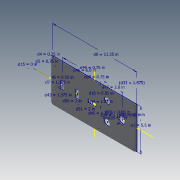
# Autodesk Inventor part: FLUGGER SWITCH PANEL
Saved by Autodesk Inventor 2020.3 (Build 243373000, 373)
## iProperties
RuleStatus: InUse
AfterDocSave0: file://Part Number Cleaner
Created: 2020-01-25
Material: Generic
Vendor: HHMI: JRC - ID&F
Document SubType Name: Modeling
Designer: arnoldj
Density: 1 g/cm^3
Appearance: Default
DESIGN DEPARTMENT: HHMI: JRC - ID&F
ALTERED ITEM PART NUMBER: N/A
ALTERED ITEM VENDOR: N/A
ALTERED ITEM DESCRIPTION: N/A
Author: arnoldj
Revision Number: 0
Autodesk Inventor part; units mm, degrees
ref_plane "YZ Plane" through (0, 0, 0) normal (1, 0, 0) x (0, 1, 0)
ref_plane "XZ Plane" through (0, 0, 0) normal (0, 1, 0) x (-1, 0, 0)
ref_plane "XY Plane" through (0, 0, 0) normal (0, 0, 1) x (1, 0, 0)
sketch "Sketch1" plane through (0, 0, 0) normal (0, 0, 1) x (1, 0, 0)
  line L0 (0, 97.79) -> (0, -97.79) projected
  line L1 (-200.025, 0) -> (200.025, 0) projected
  line L2 (142.875, -69.85) -> (-142.875, -69.85)
  line L3 (-142.875, -69.85) -> (-142.875, 69.85)
  line L4 (-142.875, 69.85) -> (142.875, 69.85)
  line L5 (142.875, 69.85) -> (142.875, -69.85)
  line L6 (142.875, -69.85) -> (-142.875, 69.85) construction
  line L7 (-142.875, -69.85) -> (142.875, 69.85) construction
  line L8 (-136.525, -63.5) -> (136.525, -63.5) construction
  line L9 (136.525, -63.5) -> (136.525, 63.5) construction
  line L10 (136.525, 63.5) -> (-136.525, 63.5) construction
  line L11 (-136.525, 63.5) -> (-136.525, -63.5) construction
  line L12 (-136.525, -63.5) -> (136.525, 63.5) construction
  line L13 (136.525, -63.5) -> (-136.525, 63.5) construction
  line L14 (-100.965, -14.2875) -> (-114.935, -14.2875)
  line L15 (-114.935, -14.2875) -> (-114.935, 14.2875)
  line L16 (-114.935, 14.2875) -> (-100.965, 14.2875)
  line L17 (-100.965, 14.2875) -> (-100.965, -14.2875)
  line L18 (-100.965, -14.2875) -> (-114.935, 14.2875) construction
  line L19 (-114.935, -14.2875) -> (-100.965, 14.2875) construction
  circle A0 centre (44.45, 31.75) radius 10.795
  circle A1 centre (44.45, -31.75) radius 10.795
  circle A2 centre (95.25, 0) radius 11.303
  circle A3 centre (95.25, 0) radius 30 construction
  line L20 (-64.135, -14.2875) -> (-50.165, -14.2875)
  line L21 (-50.165, -14.2875) -> (-50.165, 14.2875)
  line L22 (-50.165, 14.2875) -> (-64.135, 14.2875)
  line L23 (-64.135, 14.2875) -> (-64.135, -14.2875)
  line L24 (-64.135, -14.2875) -> (-50.165, 14.2875) construction
  line L25 (-50.165, -14.2875) -> (-64.135, 14.2875) construction
  line L26 (7.9375, -6.985) -> (-20.6375, -6.985)
  line L27 (-20.6375, -6.985) -> (-20.6375, 6.985)
  line L28 (-20.6375, 6.985) -> (7.9375, 6.985)
  line L29 (7.9375, 6.985) -> (7.9375, -6.985)
  line L30 (7.9375, -6.985) -> (-20.6375, 6.985) construction
  line L31 (-20.6375, -6.985) -> (7.9375, 6.985) construction
  point P0 (0, 0)
  point P1 (-107.95, 0)
  point P2 (95.25, 14.732)
  point P3 (95.25, -14.732)
  point P4 (-19.05, 63.5)
  point P5 (-19.05, -63.5)
  point P6 (19.05, -63.5)
  point P7 (19.05, 63.5)
  point P8 (-57.15, 0)
  point P9 (-6.35, 0)
  dimension "d0" = 285.75
  dimension "d1" = 139.7
  dimension "d4" = 6.35
  dimension "d5" = 6.35
  dimension "d6" = 13.97
  dimension "d7" = 28.575
  dimension "d15" = 0
  dimension "d16" = 21.59
  dimension "d20" = 22.606
  dimension "d22" = 60
  dimension "d33" = 47.625
  dimension "d34" = 14.732
  dimension "d35" = 14.732
  dimension "d43" = 34.925
  dimension "d44" = 31.75
  dimension "d45" = 31.75
  dimension "d46" = 152.4
  dimension "d47" = 50.8
  dimension "d48" = 19.05
  dimension "d49" = 19.05
  dimension "d50" = 50.8
  dimension "d51" = 50.8
  constraints: 60 end point, 10 midpoint, 10 parallel, 7 point on line, 5 coincident, 5 horizontal, 5 perpendicular, 5 vertical alignment, 4 centre point, 4 equal length, 1 equal radius
  measures "d0" distance of L3.end L4.end
  measures "d1" distance of L4.end L2.start
  measures "d4" distance between parallel lines of L4 L10
  measures "d5" distance between parallel lines of L3 L11
  measures "d6" distance of L15.end L16.end
  measures "d7" distance of L14.end L15.end
  measures "d15" distance from line of L1 point (-107.95, 0)
  measures "d16" diameter of A0
  measures "d20" diameter of A2
  measures "d22" diameter of A3
  measures "d33" distance from line of L5 A2.centre
  measures "d34" distance of A3.centre point (95.25, 14.732)
  measures "d35" distance from line of L1 point (95.25, -14.732)
  measures "d43" distance from line of L3 point (-107.95, 0)
  measures "d44" distance from line of L1 A0.centre
  measures "d45" distance from line of L1 A1.centre
  measures "d46" horizontal distance of point (-107.95, 0) A0.centre
  measures "d47" horizontal distance of A0.centre A2.centre
  measures "d48" distance from line of point (19.05, 63.5) L0
  measures "d49" distance from line of point (-19.05, 63.5) L0
  measures "d50" distance of point (-57.15, 0) point (-107.95, 0)
  measures "d51" distance of point (-57.15, 0) point (-6.35, 0)
extrude "Extrusion1" add sketch "Sketch1" along normal blind 3.175 contours L4 L5 L1 A2 L29 L28 L0 | L0 L28 L27 L1 L21 L22 L23 L17 L16 L15 L3 L4 | L1 L15 L14 L17 L23 L20 L21 L27 L26 L0 L2 L3 | L5 L2 L0 L26 L29 L1 A2
hole "Hole1" at (-136.525, 63.5, 0) at (-136.525, -63.5, 0) at (136.525, 63.5, 0) at (136.525, -63.5, 0) at (19.05, -63.5, 0) at (-19.05, 63.5, 0) at (19.05, 63.5, 0) at (-19.05, -63.5, 0) direction (0, 0, 1) diameter 5.08 end through all
fillet "Fillet1" radius 6.35 4 edges at (142.875, -69.85, 1.5875) (142.875, 69.85, 1.5875) (-142.875, -69.85, 1.5875) (-142.875, 69.85, 1.5875)
hole "Hole2" at (95.25, 14.732, 0) at (95.25, -14.732, 0) direction (0, 0, 1) diameter 3.1242 end through all
equation "\"d35\" = d34"
body "Solid1"
